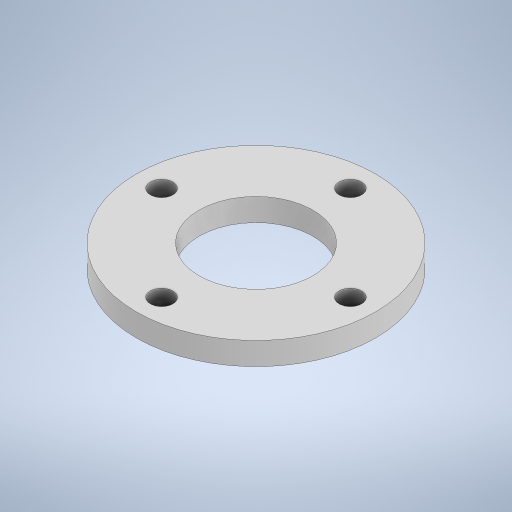
# Autodesk Inventor part: 06-01-2023 flangia DN80
Saved by Autodesk Inventor 2023 (Build 270158000, 158)
## iProperties
Created: 2023-06-01
Part Number: 06-01-2023 flangia DN80
Material: Generico
Document SubType Name: Modeling
Designer: Admin
Density: 1 g/cm^3
Appearance: Default
Author: Admin
Autodesk Inventor part; units mm, degrees
ref_plane "YZ Plane" through (0, 0, 0) normal (1, 0, 0) x (0, 1, 0)
ref_plane "XZ Plane" through (0, 0, 0) normal (0, 1, 0) x (-1, 0, 0)
ref_plane "XY Plane" through (0, 0, 0) normal (0, 0, 1) x (1, 0, 0)
sketch "Schizzo1" plane through (0, 0, 0) normal (0, 1, 0) x (-1, 0, 0)
  circle A0 centre (0, 0) radius 95
  circle A1 centre (0, 0) radius 45.25
  circle A2 centre (0, 0) radius 75 construction
  circle A3 centre (0, 75) radius 9
  circle A4 centre (-75, 0) radius 9
  circle A5 centre (0, -75) radius 9
  circle A6 centre (75, 0) radius 9
  dimension "d2" = 150
  dimension "d0" = 190
  dimension "d1" = 90.5
  dimension "d3" = 18
  dimension "d6" = 360
  constraints: 6 centre point, 3 coincident, 2 vertical alignment, 11 other
  measures "d0" diameter of A0
  measures "d1" diameter of A1
  measures "d3" diameter of A3
extrude "Estrusione1" add sketch "Schizzo1" along normal blind 18
